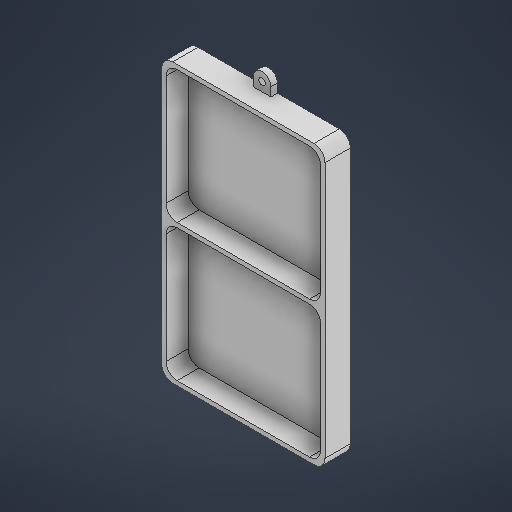
# Autodesk Inventor part: box store
Saved by Autodesk Inventor 2026.1 (Build 301233000, 233)
## iProperties
Created: 2026-03-08
Part Number: box store
Material: Generic
Document SubType Name: Modeling
Designer: momen
Density: 1 g/cm^3
Appearance: Default
Author: momen
Autodesk Inventor part; units mm, degrees
ref_plane "YZ Plane" through (0, 0, 0) normal (1, 0, 0) x (0, 1, 0)
ref_plane "XZ Plane" through (0, 0, 0) normal (0, 1, 0) x (-1, 0, 0)
ref_plane "XY Plane" through (0, 0, 0) normal (0, 0, 1) x (1, 0, 0)
sketch "Sketch1" plane through (0, 0, 0) normal (0, 0, 1) x (1, 0, 0)
  line L0 (-37, -63) -> (37, -63)
  line L1 (37, -63) -> (37, 63)
  line L2 (37, 63) -> (-37, 63)
  line L3 (-37, 63) -> (-37, -63)
  line L4 (-37, -63) -> (37, 63) construction
  line L5 (37, -63) -> (-37, 63) construction
  point P0 (0, 0)
  dimension "d0" = 74
  dimension "d1" = 126
  constraints: 12 end point, 2 midpoint, 2 parallel, 1 horizontal, 1 perpendicular
  measures "d0" distance of L2.end L1.end
  measures "d1" distance of L1.end L0.end
extrude "Extrusion1" add sketch "Sketch1" along normal blind 1.5
sketch "Sketch2" plane through (0, 0, 1.5) normal (0, 0, 1) x (1, 0, 0)
  line L0 (37, -63) -> (37, 63) projected
  line L1 (-37, -63) -> (37, -63)
  line L2 (37, -63) -> (37, 63)
  line L3 (37, 63) -> (-37, 63)
  line L4 (-37, 63) -> (-37, -63)
  line L5 (-37, -63) -> (37, 63) construction
  line L6 (37, -63) -> (-37, 63) construction
  line L7 (-35, -61) -> (35, -61)
  line L8 (35, -61) -> (35, 61)
  line L9 (35, 61) -> (-35, 61)
  line L10 (-35, 61) -> (-35, -61)
  line L11 (-35, -61) -> (35, 61) construction
  line L12 (35, -61) -> (-35, 61) construction
  line L13 (-35, -1) -> (35, -1)
  line L14 (35, -1) -> (35, 1)
  line L15 (35, 1) -> (-35, 1)
  line L16 (-35, 1) -> (-35, -1)
  line L17 (-35, -1) -> (35, 1) construction
  line L18 (35, -1) -> (-35, 1) construction
  point P0 (0, 0)
  dimension "d4" = 70
  dimension "d5" = 122
  dimension "d6" = 2
  constraints: 36 end point, 6 midpoint, 6 parallel, 3 horizontal, 3 perpendicular, 1 point on line
  measures "d4" distance of L9.end L8.end
  measures "d5" distance of L8.end L7.end
  measures "d6" distance of L14.end L13.end
extrude "Extrusion2" add sketch "Sketch2" along normal blind 10 contours L1 L4 L3 L0 | L10 L15 L8 L13
fillet "Fillet1" radius 5 12 edges at (37, 63, 5.75) (-37, 63, 5.75) (37, -63, 5.75) (-37, -63, 5.75) (-35, 61, 6.5) (35, 61, 6.5) (35, 1, 6.5) (35, -1, 6.5) (-35, 1, 6.5) (-35, -1, 6.5) (-35, -61, 6.5) (35, -61, 6.5)
sketch "Sketch3" plane through (0, 0, 0) normal (0, 0, -1) x (-1, 0, 0)
  line L0 (-32, 63) -> (32, 63) projected
  line L1 (0, 63) -> (0, 71)
  circle A0 centre (0, 67) radius 4
  circle A1 centre (0, 67) radius 1.5
  line L2 (-4, 67) -> (4, 67)
  line L3 (4, 67) -> (4, 63)
  line L4 (-4, 67) -> (-4, 63)
  line L5 (-53.0047, 0) -> (53.0047, 0)
  line L6 (-30, 1) -> (30, 1) projected
  line L7 (0, -63) -> (0, -71)
  circle A2 centre (0, -67) radius 4
  circle A3 centre (0, -67) radius 1.5
  line L8 (-4, -67) -> (4, -67)
  line L9 (4, -67) -> (4, -63)
  line L10 (-4, -67) -> (-4, -63)
  line L11 (-30, -1) -> (30, -1)
  line L12 (4, -63) -> (-4, -63)
  line L13 (32, -63) -> (-32, -63) projected
  point P0 (0, 0)
  dimension "d11" = 8
  dimension "d10" = 8
  dimension "d12" = 3
  constraints: 22 end point, 11 symmetric about line, 5 midpoint, 3 vertical, 2 centre point, 2 coincident, 2 horizontal, 2 parallel, 2 point on line, 1 collinear, 1 perpendicular, 7 other
  measures "d10" distance of L1.start L1.end
  measures "d12" diameter of A1
extrude "Extrusion3" add sketch "Sketch3" against normal blind 3 contours L4 A0 L0 | A0 L3 L0 | A0 L2 A1 L1 | L1 A1 L2 A0 | A0 L1 A1 L2 | L2 A1 L1 A0 | A2 L8 A3 L7 | L12 L9 A2 | L7 A3 L8 A2 | A2 L10 L12 | A2 L7 A3 L8 | L8 A3 L7 A2
body "Solid1"
